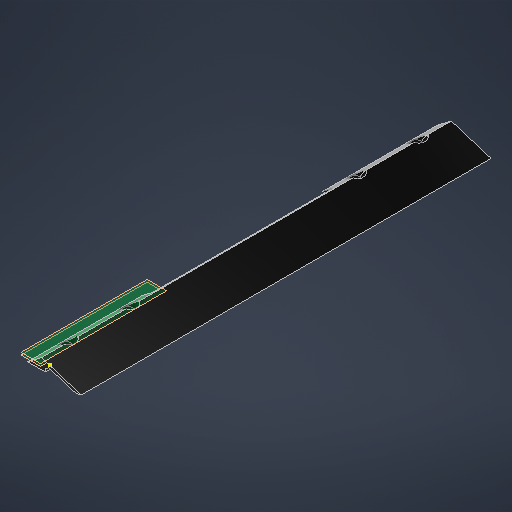
# Autodesk Inventor part: przódv3
Saved by Autodesk Inventor 2026.2 (Build 302298010, 298A)
## iProperties
Created: 2026-05-13
Part Number: przódv3
Material: Tworzywo sztuczne PET
Document SubType Name: Modeling
Designer: karol
Density: 1.541 g/cm^3
Appearance: Poliwęglan — przezroczysty
Author: karol
Autodesk Inventor part; units mm, degrees
ref_plane "YZ Plane" through (0, 0, 0) normal (1, 0, 0) x (0, 1, 0)
ref_plane "XZ Plane" through (0, 0, 0) normal (0, 1, 0) x (-1, 0, 0)
ref_plane "XY Plane" through (0, 0, 0) normal (0, 0, 1) x (1, 0, 0)
sketch "Sketch1" plane through (0, 0, 0) normal (0, 0, 1) x (1, 0, 0)
  line L0 (0.12589, -2.059002) -> (22.818207, -5.808501)
  line L1 (22.818207, -5.808501) -> (24.12238, 2.084479)
  line L2 (11.296288, 4.203761) -> (24.12238, 2.084479)
  line L3 (11.296288, 4.203761) -> (0.637289, 1.036033)
  line L4 (0.637289, 1.036033) -> (0.12589, -2.059002)
  line L5 (0, 0) -> (0, 2)
  line L6 (0, 2) -> (-6.5, 2)
  line L7 (-6.5, 0) -> (-6.5, 2)
  line L8 (0, 0) -> (-6.5, 0)
  line L9 (-6.5, 2) -> (0, 2)
  line L10 (-6.5, 2) -> (0, 2)
  line L11 (0, 2) -> (0, 3.5)
  line L12 (0, 3.5) -> (11.296288, 4.203761)
  line L13 (-2.763296, 4.833668) -> (11.202838, 5.703761)
  line L14 (11.202838, 5.703761) -> (11.296288, 4.203761)
  line L15 (-2.763296, 4.833668) -> (-6.5, 2)
  dimension "d0" = 1.5
  dimension "d1" = 1.5
  dimension "d2" = 4.68963
  constraints: 14 end point, 3 perpendicular, 1 horizontal, 1 parallel
  measures "d0" distance of L5.end L11.end
  measures "d1" vertical distance of L13.end L2.start
  measures "d2" distance of L13.start L6.end
sketch "Sketch1 outline for Extrusion1" plane through (0, 0, 0) normal (0, 0, 1) x (1, 0, 0)
  line L0 (-2.763296, 4.833668) -> (-6.5, 2)
  line L1 (11.202838, 5.703761) -> (-2.763296, 4.833668)
  line L2 (11.296288, 4.203761) -> (11.202838, 5.703761)
  line L3 (0, 3.5) -> (11.296288, 4.203761)
  line L4 (0, 2) -> (0, 3.5)
  line L5 (-6.5, 2) -> (0, 2)
extrude "Extrusion1" add sketch "Sketch1 outline for Extrusion1" against normal blind 50
sketch "Sketch2" plane through (0, 0, -50) normal (0, 0, -1) x (-1, 0, 0)
  line L0 (2.763296, 4.833668) -> (-11.202838, 5.703761)
  line L1 (-11.202838, 5.703761) -> (-5.214448, 5.330683)
  line L2 (-11.202838, 5.703761) -> (-11.296288, 4.203761)
  line L3 (-11.202838, 5.703761) -> (-11.296288, 4.203761)
  line L4 (-11.296288, 4.203761) -> (-5.307898, 3.830683)
  line L5 (-5.307898, 3.830683) -> (-5.214448, 5.330683)
  point P0 (0, 0)
  dimension "d5" = 6
  dimension "d6" = 6
  constraints: 8 end point, 1 collinear, 1 perpendicular, 1 point on line
  measures "d5" distance of L0.end L1.end
  measures "d6" distance of L2.end L4.end
sketch "Sketch2 outline for Extrusion2" plane through (0, 0, -50) normal (0, 0, -1) x (-1, 0, 0)
  line L0 (-11.296288, 4.203761) -> (-5.307898, 3.830683)
  line L1 (-11.202838, 5.703761) -> (-11.296288, 4.203761)
  line L2 (-5.214448, 5.330683) -> (-11.202838, 5.703761)
  line L3 (-5.307898, 3.830683) -> (-5.214448, 5.330683)
extrude "Extrusion2" add sketch "Sketch2 outline for Extrusion2" along normal blind 50
sketch "Sketch3" plane through (0, 0, -100) normal (0, 0, -1) x (-1, 0, 0)
  line L0 (-5.307898, 3.830683) -> (-5.214448, 5.330683)
  line L1 (-5.214448, 5.330683) -> (-11.202838, 5.703761)
  line L2 (-11.202838, 5.703761) -> (-11.296288, 4.203761)
  line L3 (-11.296288, 4.203761) -> (-5.307898, 3.830683)
  line L4 (-5.214448, 5.330683) -> (-5.307898, 3.830683)
  line L5 (-5.307898, 3.830683) -> (0, 3.5)
  line L6 (0, 3.5) -> (0, 2)
  line L7 (0, 2) -> (6.5, 2)
  line L8 (6.5, 2) -> (2.763296, 4.833668)
  line L9 (2.763296, 4.833668) -> (-5.214448, 5.330683)
  point P0 (0, 0)
sketch "Sketch3 outline for Extrusion3" plane through (0, 0, -100) normal (0, 0, -1) x (-1, 0, 0)
  line L0 (-5.307898, 3.830683) -> (0, 3.5)
  line L1 (-11.296288, 4.203761) -> (-5.307898, 3.830683)
  line L2 (-11.202838, 5.703761) -> (-11.296288, 4.203761)
  line L3 (-5.214448, 5.330683) -> (-11.202838, 5.703761)
  line L4 (2.763296, 4.833668) -> (-5.214448, 5.330683)
  line L5 (6.5, 2) -> (2.763296, 4.833668)
  line L6 (0, 2) -> (6.5, 2)
  line L7 (0, 3.5) -> (0, 2)
extrude "Extrusion3" add sketch "Sketch3 outline for Extrusion3" along normal blind 50
sketch "Sketch4" plane through (0, 0, 0) normal (0, 0, 1) x (1, 0, 0)
  line L0 (0.12589, -2.059002) -> (22.818207, -5.808501)
  line L1 (22.818207, -5.808501) -> (24.12238, 2.084479)
  line L2 (11.296288, 4.203761) -> (24.12238, 2.084479)
  line L3 (11.296288, 4.203761) -> (0.637289, 1.036033)
  line L4 (0.637289, 1.036033) -> (0.12589, -2.059002)
  line L5 (15.987807, 3.428571) -> (5.162143, 5.327424)
  line L6 (-2.763296, 4.833668) -> (11.202838, 5.703761)
  line L7 (-6.5, 2) -> (0, 2)
  line L8 (0, 2) -> (0, 3.5)
  line L9 (0, 3.5) -> (11.296288, 4.203761)
  line L10 (11.296288, 4.203761) -> (11.202838, 5.703761)
  line L11 (11.202838, 5.703761) -> (-2.763296, 4.833668)
  line L12 (-2.763296, 4.833668) -> (-6.5, 2)
  point P0 (0, 0)
  point P1 (11.293282, 4.252005)
  constraints: 2 end point, 2 point on line
sketch "Sketch4 outline for Extrusion4" plane through (0, 0, 0) normal (0, 0, 1) x (1, 0, 0)
  line L0 (11.293282, 4.252005) -> (11.202838, 5.703761)
  line L1 (5.162143, 5.327424) -> (11.293282, 4.252005)
  line L2 (11.202838, 5.703761) -> (5.162143, 5.327424)
extrude "Extrusion4" cut sketch "Sketch4 outline for Extrusion4" against normal blind 150
sketch "Sketch5" plane through (0, 0, 0) normal (0, 0, 1) x (1, 0, 0)
  line L0 (11.293282, 4.252005) -> (5.162143, 5.327424)
  line L1 (5.162143, 5.327424) -> (-2.763296, 4.833668)
  line L2 (-2.763296, 4.833668) -> (-6.5, 2)
  line L3 (-6.5, 2) -> (0, 2)
  line L4 (0, 2) -> (0, 3.5)
  line L5 (0, 3.5) -> (11.296288, 4.203761)
  line L6 (11.296288, 4.203761) -> (11.293282, 4.252005)
  line L7 (11.296288, 4.203761) -> (5.162143, 5.327424)
  line L8 (5.162143, 5.327424) -> (4.88312, 3.804219)
  line L9 (4.88312, 3.804219) -> (8.229216, 3.191275)
  line L10 (8.229216, 3.191275) -> (11.296288, 4.203761)
  line L11 (8.229216, 3.191275) -> (11.296288, 4.203761)
  point P0 (0, 0)
  constraints: 10 end point, 2 perpendicular, 1 collinear, 1 point on line
sketch "Sketch5 outline for Extrusion5" plane through (0, 0, 0) normal (0, 0, 1) x (1, 0, 0)
  line L0 (8.229216, 3.191275) -> (11.296288, 4.203761)
  line L1 (4.88312, 3.804219) -> (8.229216, 3.191275)
  line L2 (11.296288, 4.203761) -> (4.88312, 3.804219)
extrude "Extrusion5" add sketch "Sketch5 outline for Extrusion5" against normal blind 50
sketch "Sketch6" plane through (0, 0, -150) normal (0, 0, -1) x (-1, 0, 0)
  line L0 (-5.162143, 5.327424) -> (-5.215231, 5.318113)
  line L1 (-5.215231, 5.318113) -> (-5.307898, 3.830683)
  line L2 (-11.296288, 4.203761) -> (-5.307898, 3.830683)
  line L3 (-11.296288, 4.203761) -> (-8.229216, 3.191275)
  line L4 (-8.229216, 3.191275) -> (-4.88312, 3.804219)
  line L5 (-4.88312, 3.804219) -> (0, 3.5)
  line L6 (0, 3.5) -> (0, 2)
  line L7 (0, 2) -> (6.5, 2)
  line L8 (6.5, 2) -> (2.763296, 4.833668)
  line L9 (2.763296, 4.833668) -> (-5.162143, 5.327424)
  line L10 (-8.229216, 3.191275) -> (-4.88312, 3.804219)
  line L11 (-11.296288, 4.203761) -> (-8.229216, 3.191275)
  point P0 (0, 0)
  constraints: 4 end point, 2 collinear
sketch "Sketch6 outline for Extrusion6" plane through (0, 0, -150) normal (0, 0, -1) x (-1, 0, 0)
  line L0 (-5.307898, 3.830683) -> (-11.296288, 4.203761)
  line L1 (-5.215231, 5.318113) -> (-5.307898, 3.830683)
  line L2 (-5.162143, 5.327424) -> (-5.215231, 5.318113)
  line L3 (2.763296, 4.833668) -> (-5.162143, 5.327424)
  line L4 (6.5, 2) -> (2.763296, 4.833668)
  line L5 (0, 2) -> (6.5, 2)
  line L6 (0, 3.5) -> (0, 2)
  line L7 (-4.88312, 3.804219) -> (0, 3.5)
  line L8 (-8.229216, 3.191275) -> (-4.88312, 3.804219)
  line L9 (-11.296288, 4.203761) -> (-8.229216, 3.191275)
extrude "Extrusion6" add sketch "Sketch6 outline for Extrusion6" against normal blind 50
sketch "Sketch8" plane through (0, 0, 0) normal (0, 0, 1) x (1, 0, 0)
  line L0 (0, 3.5) -> (0, 2)
  line L1 (0, 3.001944) -> (6.912008, 3.432564)
  line L2 (8.229216, 3.191275) -> (4.88312, 3.804219)
  line L3 (5.162143, 5.327424) -> (-2.763296, 4.833668)
  line L4 (11.293282, 4.252005) -> (5.162143, 5.327424)
  line L5 (5.162143, 5.327424) -> (-2.763296, 4.833668)
  line L6 (-2.763296, 4.833668) -> (-6.5, 2)
  line L7 (-6.5, 2) -> (0, 2)
  line L8 (0, 2) -> (0, 3.5)
  line L9 (0, 3.5) -> (4.88312, 3.804219)
  line L10 (4.88312, 3.804219) -> (8.229216, 3.191275)
  line L11 (8.229216, 3.191275) -> (11.296288, 4.203761)
  line L12 (11.296288, 4.203761) -> (11.293282, 4.252005)
  point P0 (0, 0)
  dimension "d19" = 2
  constraints: 2 end point, 2 point on line, 1 parallel
  measures "d19" distance between parallel lines of L3 L1
sketch "Sketch8 outline for Extrusion8" plane through (0, 0, 0) normal (0, 0, 1) x (1, 0, 0)
  line L0 (4.88312, 3.804219) -> (0, 3.5)
  line L1 (6.912008, 3.432564) -> (4.88312, 3.804219)
  line L2 (0, 3.001944) -> (6.912008, 3.432564)
  line L3 (0, 3.5) -> (0, 3.001944)
extrude "Extrusion8" add sketch "Sketch8 outline for Extrusion8" against normal blind 50
sketch "Sketch9" plane through (0, 0, -150) normal (0, 0, -1) x (-1, 0, 0)
  line L0 (-4.88312, 3.804219) -> (0, 3.5)
  line L1 (-5.162143, 5.327424) -> (-5.215231, 5.318113)
  line L2 (-5.215231, 5.318113) -> (-5.307898, 3.830683)
  line L3 (-11.296288, 4.203761) -> (-5.307898, 3.830683)
  line L4 (-11.296288, 4.203761) -> (-8.229216, 3.191275)
  line L5 (-8.229216, 3.191275) -> (-6.912008, 3.432564)
  line L6 (-6.912008, 3.432564) -> (0, 3.001944)
  line L7 (0, 3.001944) -> (0, 2)
  line L8 (0, 2) -> (6.5, 2)
  line L9 (6.5, 2) -> (2.763296, 4.833668)
  line L10 (2.763296, 4.833668) -> (-5.162143, 5.327424)
  line L11 (-6.912008, 3.432564) -> (-4.88312, 3.804219)
  line L12 (0, 3.001944) -> (0, 3.5)
  point P0 (0, 0)
  constraints: 4 end point, 1 vertical
sketch "Sketch9 outline for Extrusion9" plane through (0, 0, -150) normal (0, 0, -1) x (-1, 0, 0)
  line L0 (-6.912008, 3.432564) -> (0, 3.001944)
  line L1 (-4.88312, 3.804219) -> (-6.912008, 3.432564)
  line L2 (0, 3.5) -> (-4.88312, 3.804219)
  line L3 (0, 3.001944) -> (0, 3.5)
extrude "Extrusion9" add sketch "Sketch9 outline for Extrusion9" against normal blind 50
sketch "Sketch10" plane through (0, 0, -150) normal (0, 0, -1) x (-1, 0, 0)
  line L0 (-5.307898, 3.830683) -> (-11.296288, 4.203761)
  line L1 (-6.912008, 3.432564) -> (-8.229216, 3.191275)
  line L2 (-11.296288, 4.203761) -> (-8.229216, 3.191275)
  line L3 (-8.229216, 3.191275) -> (-8.018718, 3.229835)
  line L4 (-8.018718, 3.229835) -> (-11.296288, 4.203761)
  point P0 (0, 0)
  dimension "d24" = 0.214
  constraints: 6 end point, 1 point on line
  measures "d24" distance of L1.end L3.end
sketch "Sketch10 outline for Extrusion10" plane through (0, 0, -150) normal (0, 0, -1) x (-1, 0, 0)
  line L0 (-11.296288, 4.203761) -> (-8.229216, 3.191275)
  line L1 (-8.018718, 3.229835) -> (-11.296288, 4.203761)
  line L2 (-8.229216, 3.191275) -> (-8.018718, 3.229835)
extrude "Extrusion10" cut sketch "Sketch10 outline for Extrusion10" against normal blind 150
sketch "Szkic11" plane through (0, 0, -100) normal (0, 0, 1) x (1, 0, 0)
  line L0 (8.018718, 3.229835) -> (11.296288, 4.203761)
  line L1 (5.307898, 3.830683) -> (11.296288, 4.203761)
  line L2 (5.307898, 3.830683) -> (5.215231, 5.318113)
  line L3 (5.215231, 5.318113) -> (5.162143, 5.327424)
  line L4 (-2.763296, 4.833668) -> (5.162143, 5.327424)
  line L5 (-6.5, 2) -> (-2.763296, 4.833668)
  line L6 (0, 2) -> (-6.5, 2)
  line L7 (0, 3.001944) -> (0, 2)
  line L8 (0, 3.001944) -> (6.912008, 3.432564)
  line L9 (6.912008, 3.432564) -> (8.018718, 3.229835)
  line L10 (5.215231, 5.318113) -> (5.338807, 3.334553)
  point P0 (0, 0)
  constraints: 2 end point, 2 point on line
sketch "Szkic11 outline for Wyciągnięcie proste11" plane through (0, 0, -100) normal (0, 0, 1) x (1, 0, 0)
  line L0 (5.215231, 5.318113) -> (5.162143, 5.327424)
  line L1 (5.307898, 3.830683) -> (5.215231, 5.318113)
  line L2 (5.338807, 3.334553) -> (5.307898, 3.830683)
  line L3 (0, 3.001944) -> (5.338807, 3.334553)
  line L4 (0, 2) -> (0, 3.001944)
  line L5 (-6.5, 2) -> (0, 2)
  line L6 (-2.763296, 4.833668) -> (-6.5, 2)
  line L7 (5.162143, 5.327424) -> (-2.763296, 4.833668)
extrude "Wyciągnięcie proste11" cut sketch "Szkic11 outline for Wyciągnięcie proste11" against normal blind 8
sketch "Szkic12" plane through (0, 0, -50) normal (0, 0, -1) x (-1, 0, 0)
  line L0 (-11.296288, 4.203761) -> (-8.018718, 3.229835)
  line L1 (-8.018718, 3.229835) -> (-6.912008, 3.432564)
  line L2 (-6.912008, 3.432564) -> (0, 3.001944)
  line L3 (0, 3.001944) -> (0, 2)
  line L4 (0, 2) -> (6.5, 2)
  line L5 (6.5, 2) -> (2.763296, 4.833668)
  line L6 (2.763296, 4.833668) -> (-5.162143, 5.327424)
  line L7 (-5.162143, 5.327424) -> (-11.293282, 4.252005)
  line L8 (-11.293282, 4.252005) -> (-11.296288, 4.203761)
  line L9 (-5.215231, 5.318113) -> (-5.307898, 3.830683)
  line L10 (-5.215231, 5.318113) -> (-5.338807, 3.334553)
  point P0 (0, 0)
  constraints: 2 end point, 1 perpendicular, 1 point on line
sketch "Szkic12 outline for Wyciągnięcie proste12" plane through (0, 0, -50) normal (0, 0, -1) x (-1, 0, 0)
  line L0 (2.763296, 4.833668) -> (-5.162143, 5.327424)
  line L1 (6.5, 2) -> (2.763296, 4.833668)
  line L2 (0, 2) -> (6.5, 2)
  line L3 (0, 3.001944) -> (0, 2)
  line L4 (-5.338807, 3.334553) -> (0, 3.001944)
  line L5 (-5.307898, 3.830683) -> (-5.338807, 3.334553)
  line L6 (-5.215231, 5.318113) -> (-5.307898, 3.830683)
  line L7 (-5.162143, 5.327424) -> (-5.215231, 5.318113)
extrude "Wyciągnięcie proste12" cut sketch "Szkic12 outline for Wyciągnięcie proste12" against normal blind 8
sketch "Szkic13" plane through (-6.5, 2, 0) normal (0, -1, 0) x (1, 0, 0)
  circle A0 centre (3.25, -11) radius 1.55
  circle A1 centre (3.25, -33.5) radius 1.55
  circle A2 centre (3.25, -116.5) radius 1.55
  circle A3 centre (3.25, -139) radius 1.55
  line L0 (6.5, -150) -> (0, -150) projected
  line L1 (0, 0) -> (6.5, 0) projected
  line L2 (0, -108) -> (0, -150) projected
  line L3 (0, 0) -> (0, -42) projected
  dimension "d31" = 3.1
  dimension "d32" = 3.1
  dimension "d33" = 3.1
  dimension "d34" = 3.1
  dimension "d35" = 11
  dimension "d36" = 33.5
  dimension "d37" = 33.5
  dimension "d38" = 11
  dimension "d39" = 3.25
  dimension "d40" = 3.25
  dimension "d41" = 3.25
  dimension "d42" = 3.25
  constraints: 4 centre point
  measures "d31" diameter of A0
  measures "d32" diameter of A1
  measures "d33" diameter of A2
  measures "d34" diameter of A3
  measures "d35" distance from line of L0 A3.centre
  measures "d36" distance from line of L0 A2.centre
  measures "d37" distance from line of L1 A1.centre
  measures "d38" distance from line of L1 A0.centre
  measures "d39" distance from line of L2 A3.centre
  measures "d40" distance from line of L2 A2.centre
  measures "d41" distance from line of L3 A1.centre
  measures "d42" distance from line of L3 A0.centre
sketch "Szkic13 outline for Wyciągnięcie proste13" plane through (-6.5, 2, 0) normal (0, -1, 0) x (1, 0, 0)
  circle A0 centre (3.25, -139) radius 1.55
  circle A1 centre (3.25, -11) radius 1.55
  circle A2 centre (3.25, -33.5) radius 1.55
  circle A3 centre (3.25, -116.5) radius 1.55
extrude "Wyciągnięcie proste13" cut sketch "Szkic13 outline for Wyciągnięcie proste13" against normal blind 3
ref_plane "Płaszczyzna konstrukcyjna1" through (-6.5, 5, 0) normal (0, -1, 0) x (1, 0, 0)
sketch "Szkic15" plane through (-6.5, 5, 0) normal (0, -1, 0) x (1, 0, 0)
  arc A0 (3.736704, -9.528396) -> (3.736704, -12.471604) centre (3.25, -11) ccw
  arc A1 (3.736704, -32.028396) -> (3.736704, -34.971604) centre (3.25, -33.5) ccw
  arc A2 (3.736704, -115.028396) -> (3.736704, -117.971604) centre (3.25, -116.5) ccw
  arc A3 (3.736704, -137.528396) -> (3.736704, -140.471604) centre (3.25, -139) ccw
  point P0 (6.5, 0)
hole "Otwór2" at (-3.25, 5, -11) at (-3.25, 5, -33.5) at (-3.25, 5, -139) at (-3.25, 5, -116.5) direction (0, -1, 0) diameter 3.1 depth 3 tip angle 118 countersink diameter 6.3 countersink angle 90
sketch "Szkic16" plane through (0, 0, 0) normal (0, 0, 1) x (1, 0, 0)
  line L0 (6.912008, 3.432564) -> (0, 3.001944)
  line L1 (11.296288, 4.203761) -> (8.018718, 3.229835)
  line L2 (6.912008, 3.432564) -> (8.018718, 3.229835)
  line L3 (8.018718, 3.229835) -> (6.912008, 3.432564)
  line L4 (13.251736, 2.742052) -> (2.458388, 0.067655)
  line L5 (6.912008, 3.432564) -> (10.897705, 2.158765)
  line L6 (-2.763296, 4.833668) -> (5.162143, 5.327424)
  line L7 (5.162143, 5.327424) -> (13.251736, 2.742052)
  line L8 (5.162143, 5.327424) -> (11.293282, 4.252005)
  line L9 (5.162143, 5.327424) -> (11.293282, 4.252005)
  line L10 (11.293282, 4.252005) -> (11.296288, 4.203761)
  line L11 (11.296288, 4.203761) -> (9.93954, 3.800605)
  line L12 (8.018718, 3.229835) -> (9.93954, 3.800605)
  line L13 (13.251736, 2.742052) -> (10.897705, 2.158765)
  point P0 (0, 0)
  constraints: 18 end point, 4 collinear, 4 point on line, 1 parallel
sketch "Szkic16 outline for Wyciągnięcie proste14" plane through (0, 0, 0) normal (0, 0, 1) x (1, 0, 0)
  line L0 (13.251736, 2.742052) -> (9.93954, 3.800605)
  line L1 (10.897705, 2.158765) -> (13.251736, 2.742052)
  line L2 (6.912008, 3.432564) -> (10.897705, 2.158765)
  line L3 (8.018718, 3.229835) -> (6.912008, 3.432564)
  line L4 (9.93954, 3.800605) -> (8.018718, 3.229835)
extrude "Wyciągnięcie proste14" add sketch "Szkic16 outline for Wyciągnięcie proste14" against normal blind 150
sketch "Szkic17" plane through (0, 0, 0) normal (0, 0, 1) x (1, 0, 0)
  line L0 (-2.763296, 4.833668) -> (5.162143, 5.327424)
  line L1 (13.251736, 2.742052) -> (9.93954, 3.800605)
  line L2 (5.162143, 5.327424) -> (9.93954, 3.800605)
  line L3 (9.93954, 3.800605) -> (11.296288, 4.203761)
  line L4 (9.93954, 3.800605) -> (11.296288, 4.203761)
  line L5 (11.296288, 4.203761) -> (11.293282, 4.252005)
  line L6 (11.296288, 4.203761) -> (11.293282, 4.252005)
  line L7 (11.293282, 4.252005) -> (5.162143, 5.327424)
  line L8 (11.293282, 4.252005) -> (5.162143, 5.327424)
  point P0 (0, 0)
  constraints: 8 end point, 4 collinear
sketch "Szkic17 outline for Wyciągnięcie proste15" plane through (0, 0, 0) normal (0, 0, 1) x (1, 0, 0)
  line L0 (5.162143, 5.327424) -> (9.93954, 3.800605)
  line L1 (11.293282, 4.252005) -> (5.162143, 5.327424)
  line L2 (11.296288, 4.203761) -> (11.293282, 4.252005)
  line L3 (9.93954, 3.800605) -> (11.296288, 4.203761)
extrude "Wyciągnięcie proste15" cut sketch "Szkic17 outline for Wyciągnięcie proste15" against normal blind 150
sketch "Szkic18" plane through (0, 0, 0) normal (0, 0, 1) x (1, 0, 0)
  line L0 (6.912008, 3.432564) -> (10.897705, 2.158765)
  line L1 (10.897705, 2.158765) -> (6.912008, 3.432564)
  line L2 (10.897705, 2.158765) -> (13.251736, 2.742052)
  line L3 (6.912008, 3.432564) -> (10.897705, 2.158765)
  line L4 (13.251736, 2.742052) -> (5.162143, 5.327424)
  line L5 (13.251736, 2.742052) -> (5.162143, 5.327424)
  line L6 (5.162143, 5.327424) -> (2.295716, 5.148845)
  line L7 (5.162143, 5.327424) -> (-2.763296, 4.833668)
  line L8 (10.897705, 2.158765) -> (1.664781, 5.109538)
  point P0 (0, 0)
  point P1 (1.664781, 5.109538)
  constraints: 10 end point, 3 collinear, 2 point on line, 1 parallel
sketch "Szkic18 outline for Wyciągnięcie proste16" plane through (0, 0, 0) normal (0, 0, 1) x (1, 0, 0)
  line L0 (10.897705, 2.158765) -> (13.251736, 2.742052)
  line L1 (6.912008, 3.432564) -> (10.897705, 2.158765)
  line L2 (1.664781, 5.109538) -> (6.912008, 3.432564)
  line L3 (2.295716, 5.148845) -> (1.664781, 5.109538)
  line L4 (5.162143, 5.327424) -> (2.295716, 5.148845)
  line L5 (13.251736, 2.742052) -> (5.162143, 5.327424)
extrude "Wyciągnięcie proste16" add sketch "Szkic18 outline for Wyciągnięcie proste16" against normal blind 150
sketch "Szkic19" plane through (0, 0, 0) normal (0, 0, 1) x (1, 0, 0)
  line L0 (5.162143, 5.327424) -> (-2.763296, 4.833668)
  line L1 (-2.763296, 4.833668) -> (-6.5, 2)
  line L2 (-6.5, 2) -> (0, 2)
  line L3 (0, 2) -> (0, 3.001944)
  line L4 (0, 3.001944) -> (6.912008, 3.432564)
  line L5 (6.912008, 3.432564) -> (10.897705, 2.158765)
  line L6 (10.897705, 2.158765) -> (13.251736, 2.742052)
  line L7 (13.251736, 2.742052) -> (5.162143, 5.327424)
  line L8 (0, 3.001944) -> (10.897705, 2.158765)
  line L9 (-2.763296, 4.833668) -> (5.162143, 5.327424)
  line L10 (5.162143, 5.327424) -> (13.251736, 2.742052)
  line L11 (0, 3.001944) -> (6.912008, 3.432564)
  point P0 (0, 0)
  constraints: 4 end point, 1 parallel, 1 point on line
sketch "Szkic19 outline for Wyciągnięcie proste17" plane through (0, 0, 0) normal (0, 0, 1) x (1, 0, 0)
  line L0 (0, 3.001944) -> (10.897705, 2.158765)
  line L1 (6.912008, 3.432564) -> (0, 3.001944)
  line L2 (10.897705, 2.158765) -> (6.912008, 3.432564)
extrude "Wyciągnięcie proste17" add sketch "Szkic19 outline for Wyciągnięcie proste17" against normal blind 150
sketch "Szkic20" plane through (0, 0, 0) normal (0, 0, 1) x (1, 0, 0)
  line L0 (-2.763296, 4.833668) -> (5.162143, 5.327424)
  line L1 (-2.763296, 4.833668) -> (9.732218, 3.866863)
  line L2 (5.162143, 5.327424) -> (13.251736, 2.742052)
  line L3 (0, 3.001944) -> (10.897705, 2.158765)
  point P0 (0, 0)
  constraints: 2 end point, 1 parallel, 1 point on line
sketch "Szkic20 outline for Wyciągnięcie proste18" plane through (0, 0, 0) normal (0, 0, 1) x (1, 0, 0)
  line L0 (5.162143, 5.327424) -> (-2.763296, 4.833668)
  line L1 (9.732218, 3.866863) -> (5.162143, 5.327424)
  line L2 (-2.763296, 4.833668) -> (9.732218, 3.866863)
extrude "Wyciągnięcie proste18" cut sketch "Szkic20 outline for Wyciągnięcie proste18" against normal blind 150
sketch "Szkic21" plane through (0, 3.001944, -42) normal (-0.0621796, 0.998065, 0) x (0.998065, 0.0621796, 0)
  line L0 (5.349158, 66) -> (0, 66)
  line L1 (0, 0) -> (0, 66)
  line L2 (0, 0) -> (5.349158, 0)
  line L3 (5.349158, 0) -> (5.349158, 8)
  line L4 (6.925409, 8) -> (5.349158, 8)
  line L5 (6.925409, 58) -> (6.925409, 8)
  line L6 (5.349158, 58) -> (6.925409, 58)
  line L7 (5.349158, 58) -> (5.349158, 66)
  line L8 (0, 66) -> (-0.062301, 66)
  line L9 (-0.062301, 66) -> (5.349158, 66)
  line L10 (5.349158, 66) -> (5.349158, 0)
  line L11 (5.349158, 0) -> (-0.062301, 0)
  line L12 (-0.062301, 0) -> (-0.062301, 66)
  point P0 (-0.18666, -42)
  constraints: 8 end point, 2 parallel, 1 horizontal, 1 perpendicular
sketch "Szkic21 outline for Wyciągnięcie proste19" plane through (0, 3.001944, -42) normal (-0.0621796, 0.998065, 0) x (0.998065, 0.0621796, 0)
  line L0 (-0.062301, 66) -> (-0.062301, 0)
  line L1 (0, 66) -> (-0.062301, 66)
  line L2 (5.349158, 66) -> (0, 66)
  line L3 (5.349158, 58) -> (5.349158, 66)
  line L4 (5.349158, 8) -> (5.349158, 58)
  line L5 (5.349158, 0) -> (5.349158, 8)
  line L6 (0, 0) -> (5.349158, 0)
  line L7 (-0.062301, 0) -> (0, 0)
extrude "Wyciągnięcie proste19" cut sketch "Szkic21 outline for Wyciągnięcie proste19" against normal blind 150
sketch "Szkic22" plane through (9.732218, 3.866863, 0) normal (0.0771416, 0.9970201, 0) x (0.9970201, -0.0771416, 0)
  line L0 (-5.53054, 42) -> (-5.53054, 108)
  line L1 (-5.53054, 108) -> (-3.53054, 108)
  line L2 (-3.53054, 108) -> (-3.53054, 42)
  line L3 (-3.53054, 42) -> (-5.53054, 42)
  line L4 (-5.53054, 42) -> (-5.53054, 108)
  point P0 (-9.404922, 0)
  dimension "d72" = 2
  constraints: 8 end point, 2 parallel, 1 horizontal, 1 perpendicular
  measures "d72" distance of L2.end L3.end
sketch "Szkic22 outline for Wyciągnięcie proste20" plane through (9.732218, 3.866863, 0) normal (0.0771416, 0.9970201, 0) x (0.9970201, -0.0771416, 0)
  line L0 (-5.53054, 42) -> (-3.53054, 42)
  line L1 (-5.53054, 108) -> (-5.53054, 42)
  line L2 (-3.53054, 108) -> (-5.53054, 108)
  line L3 (-3.53054, 42) -> (-3.53054, 108)
extrude "Wyciągnięcie proste20" cut sketch "Szkic22 outline for Wyciągnięcie proste20" against normal blind 150
sketch "Szkic23" plane through (6.212199, 4.139215, -108) normal (-0.9970201, 0.0771416, 0) x (0, 0, 1)
  line L0 (66, -1.6131) -> (0, -1.6131)
  line L1 (66, 0) -> (66, -1.6131)
  line L2 (0, 0) -> (66, 0)
  line L3 (0, 0) -> (0, -1.6131)
  line L4 (58, -0.472751) -> (8, -0.472751)
  line L5 (58, -0.756136) -> (58, -0.472751)
  line L6 (8, -0.756136) -> (58, -0.756136)
  line L7 (8, -0.472751) -> (8, -0.756136)
  line L8 (58, -0.472751) -> (8, -0.472751)
  point P0 (108, -4.606099)
sketch "Szkic23 outline for Wyciągnięcie proste21" plane through (6.212199, 4.139215, -108) normal (-0.9970201, 0.0771416, 0) x (0, 0, 1)
  line L0 (0, 0) -> (0, -1.6131)
  line L1 (66, 0) -> (0, 0)
  line L2 (66, -1.6131) -> (66, 0)
  line L3 (0, -1.6131) -> (66, -1.6131)
extrude "Wyciągnięcie proste21" cut sketch "Szkic23 outline for Wyciągnięcie proste21" against normal blind 0.8
sketch "Sketch24" plane through (0, 0, -150) normal (0, 0, -1) x (-1, 0, 0)
  line L0 (2.763296, 4.833668) -> (0.445653, 4.654347)
  line L1 (2.763296, 4.833668) -> (6.5, 2)
  line L2 (2.763296, 4.833668) -> (6.5, 2)
  line L3 (-13.251736, 2.742052) -> (-25.966849, 0.035409)
  line L4 (-25.966849, 0.035409) -> (1.997331, 5.988093)
  line L5 (6.5, 2) -> (1.406755, 5.862378)
  line L6 (-9.732218, 3.866863) -> (-13.251736, 2.742052)
  line L7 (-13.251736, 2.742052) -> (-9.732218, 3.866863)
  line L8 (-9.732218, 3.866863) -> (-6.960049, 4.081352)
  line L9 (-6.960049, 4.081352) -> (2.763296, 4.833668)
  line L10 (-10.897705, 2.158765) -> (0, 3.001944)
  line L11 (-10.897705, 2.158765) -> (2.523294, 5.015669)
  line L12 (-10.897705, 2.158765) -> (0, 3.001944)
  line L13 (0, 3.001944) -> (-1.52038, 4.1549)
  point P0 (0, 0)
  point P1 (-13.251736, 2.742052)
  constraints: 20 end point, 6 point on line, 4 collinear, 2 parallel, 3 other
sketch "Sketch24 outline for Extrusion22" plane through (0, 0, -150) normal (0, 0, -1) x (-1, 0, 0)
  line L0 (-6.960049, 4.081352) -> (-9.732218, 3.866863)
  line L1 (-13.251736, 2.742052) -> (-6.960049, 4.081352)
  line L2 (-9.732218, 3.866863) -> (-13.251736, 2.742052)
  line L3 (0, 3.001944) -> (-1.52038, 4.1549)
  line L4 (-10.897705, 2.158765) -> (0, 3.001944)
  line L5 (-1.52038, 4.1549) -> (-10.897705, 2.158765)
extrude "Extrusion22" cut sketch "Sketch24 outline for Extrusion22" against normal blind 150
sketch "Sketch24 outline for Extrusion23" plane through (0, 0, -150) normal (0, 0, -1) x (-1, 0, 0)
  line L0 (2.763296, 4.833668) -> (1.406755, 5.862378)
  line L1 (0.445653, 4.654347) -> (2.763296, 4.833668)
  line L2 (-6.960049, 4.081352) -> (0.445653, 4.654347)
  line L3 (1.406755, 5.862378) -> (-6.960049, 4.081352)
extrude "Extrusion23" add sketch "Sketch24 outline for Extrusion23" against normal blind 150
sketch "Sketch25" plane through (0, 0, -150) normal (0, 0, -1) x (-1, 0, 0)
  line L0 (4.653847, 3.4) -> (1.7, 3.4)
  line L1 (1.406755, 5.862378) -> (-13.251736, 2.742052)
  line L2 (-13.251736, 2.742052) -> (-10.897705, 2.158765)
  line L3 (-10.897705, 2.158765) -> (-1.52038, 4.1549)
  line L4 (-1.52038, 4.1549) -> (0, 3.001944)
  line L5 (0, 3.001944) -> (0, 2)
  line L6 (0, 2) -> (6.5, 2)
  line L7 (6.5, 2) -> (1.406755, 5.862378)
  line L8 (-1.52038, 4.1549) -> (1.406755, 5.862378)
  point P0 (0, 0)
  constraints: 2 end point
sketch "Sketch25 outline for Extrusion24" plane through (0, 0, -150) normal (0, 0, -1) x (-1, 0, 0)
  line L0 (1.406755, 5.862378) -> (-13.251736, 2.742052)
  line L1 (-1.52038, 4.1549) -> (1.406755, 5.862378)
  line L2 (-10.897705, 2.158765) -> (-1.52038, 4.1549)
  line L3 (-13.251736, 2.742052) -> (-10.897705, 2.158765)
extrude "Extrusion24" add sketch "Sketch25 outline for Extrusion24" against normal blind 150
sketch "Szkic26" plane through (0, 0, 0) normal (0, 0, 1) x (1, 0, 0)
  line L0 (13.135536, 1.273992) -> (2.200131, -0.742362)
  line L1 (22.772476, -1.396098) -> (13.135536, 1.273992)
  line L2 (0, 3.001944) -> (1.52038, 4.1549)
  line L3 (1.52038, 4.1549) -> (10.897705, 2.158765)
  line L4 (10.897705, 2.158765) -> (13.251736, 2.742052)
  line L5 (13.251736, 2.742052) -> (-1.406755, 5.862378)
  line L6 (-1.406755, 5.862378) -> (-6.5, 2)
  line L7 (-6.5, 2) -> (0, 2)
  line L8 (0, 2) -> (0, 3.001944)
  line L9 (0, 3.001944) -> (1.52038, 4.1549)
  line L10 (1.52038, 4.1549) -> (10.897705, 2.158765)
  line L11 (10.897705, 2.158765) -> (13.251736, 2.742052)
  line L12 (13.251736, 2.742052) -> (-1.406755, 5.862378)
  line L13 (-1.406755, 5.862378) -> (13.135536, 1.273992)
  line L14 (1.273897, 3.967983) -> (11.037958, 0.887225)
  point P0 (0, 0)
  point P1 (5.86439, 3.568185)
  point P2 (9.156947, 2.529317)
  dimension "d84" = 1
  constraints: 8 end point, 2 point on line, 1 midpoint, 1 parallel, 5 other
  measures "d84" distance from line of point (5.864, 3.568) L14
sketch "Szkic26 outline for Wyciągnięcie proste25" plane through (0, 0, 0) normal (0, 0, 1) x (1, 0, 0)
  line L0 (-1.406755, 5.862378) -> (9.156947, 2.529317)
  line L1 (13.251736, 2.742052) -> (-1.406755, 5.862378)
  line L2 (10.897705, 2.158765) -> (13.251736, 2.742052)
  line L3 (9.156947, 2.529317) -> (10.897705, 2.158765)
extrude "Wyciągnięcie proste25" cut sketch "Szkic26 outline for Wyciągnięcie proste25" against normal blind 150
sketch "Szkic26 outline for Wyciągnięcie proste26" plane through (0, 0, 0) normal (0, 0, 1) x (1, 0, 0)
  line L0 (1.273897, 3.967983) -> (11.037958, 0.887225)
  line L1 (1.52038, 4.1549) -> (1.273897, 3.967983)
  line L2 (9.156947, 2.529317) -> (1.52038, 4.1549)
  line L3 (13.135536, 1.273992) -> (9.156947, 2.529317)
  line L4 (11.037958, 0.887225) -> (13.135536, 1.273992)
extrude "Wyciągnięcie proste26" add sketch "Szkic26 outline for Wyciągnięcie proste26" against normal blind 150
ref_plane "Płaszczyzna konstrukcyjna2" through (-6.5, 5.87, 0) normal (0, -1, 0) x (1, 0, 0)
sketch "Szkic27" plane through (-1.406755, 5.862378, 0) normal (0.3008978, 0.9536564, 0) x (0.9536564, -0.3008978, 0)
  point P0 (3.105538, 0)
sketch "Szkic28" plane through (-6.5, 5, 0) normal (0, -1, 0) x (1, 0, 0)
  circle A0 centre (3.25, -11) radius 1.55
  circle A1 centre (3.25, -11) radius 1.55
  circle A2 centre (3.25, -33.5) radius 1.55
  circle A3 centre (3.25, -33.5) radius 1.55
  arc A4 (1.846153, -117.15705) -> (1.846153, -115.84295) centre (3.25, -116.5) ccw
  circle A5 centre (3.25, -116.5) radius 1.55
  circle A6 centre (3.25, -139) radius 1.55
  circle A7 centre (3.25, -139) radius 1.55
  point P0 (6.5, 0)
  constraints: 4 centre point, 4 coincident
hole "Otwór3" at (-3.25, 5, -139) at (-3.25, 5, -116.5) at (-3.25, 5, -33.5) at (-3.25, 5, -11) direction (0, -1, 0) diameter 3.1 depth 3 tip angle 118 countersink diameter 6.3 countersink angle 90
sketch "Szkic29" plane through (-6.5, 5, 0) normal (0, -1, 0) x (1, 0, 0)
  circle A0 centre (3.25, -11) radius 3.15
  arc A1 (3.956043, -14.069854) -> (3.956043, -7.930146) centre (3.25, -11) ccw
  circle A2 centre (3.25, -116.5) radius 3.15
  circle A3 centre (3.25, -33.5) radius 3.15
  circle A4 centre (3.25, -139) radius 3.15
  arc A5 (3.956043, -119.569854) -> (3.956043, -113.430146) centre (3.25, -116.5) ccw
  arc A6 (3.956043, -142.069854) -> (3.956043, -135.930146) centre (3.25, -139) ccw
  arc A7 (3.956043, -36.569854) -> (3.956043, -30.430146) centre (3.25, -33.5) ccw
  point P0 (6.5, 0)
  dimension "d97" = 6.3
  dimension "d98" = 6.3
  dimension "d99" = 6.3
  dimension "d100" = 6.3
  constraints: 4 centre point, 4 concentric
  measures "d97" diameter of A0
  measures "d98" diameter of A2
  measures "d99" diameter of A3
  measures "d100" diameter of A4
sketch "Szkic29 outline for Wyciągnięcie proste27" plane through (-6.5, 5, 0) normal (0, -1, 0) x (1, 0, 0)
  circle A0 centre (3.25, -33.5) radius 3.15
  circle A1 centre (3.25, -139) radius 3.15
  circle A2 centre (3.25, -116.5) radius 3.15
  circle A3 centre (3.25, -11) radius 3.15
extrude "Wyciągnięcie proste27" cut sketch "Szkic29 outline for Wyciągnięcie proste27" against normal blind 2
body "Solid1"
